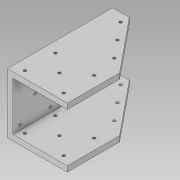
# Autodesk Inventor part: complex_cube
Saved by Autodesk Inventor 2017 (Build 210142000, 142)
## iProperties
Part Number: complex_cube
Material: Generisch
Document SubType Name: Modeling
Designer: Max
Density: 1 g/cm^3
Appearance: Vorgabe
Author: Max
Autodesk Inventor part; units mm, degrees
ref_plane "YZ Plane" through (0, 0, 0) normal (1, 0, 0) x (0, 1, 0)
ref_plane "XZ Plane" through (0, 0, 0) normal (0, 1, 0) x (-1, 0, 0)
ref_plane "XY Plane" through (0, 0, 0) normal (0, 0, 1) x (1, 0, 0)
sketch "Skizze1" plane through (0, 0, 0) normal (0, 1, 0) x (-1, 0, 0)
  line L0 (-27, 27) -> (27, 27)
  line L1 (27, 27) -> (27, -27)
  line L2 (27, -27) -> (-27, -27)
  line L3 (-27, -27) -> (-27, 27)
  line L4 (-27, 27) -> (27, -27) construction
  line L5 (27, 27) -> (-27, -27) construction
  point P0 (0, 0)
  dimension "d0" = 54
  dimension "d1" = 54
  constraints: 12 end point, 2 midpoint, 2 parallel, 1 horizontal, 1 perpendicular
  measures "d0" distance of L1.end L2.end
  measures "d1" distance of L0.end L1.end
extrude "Extrusion1" add sketch "Skizze1" along normal blind 95
sketch "Skizze2" plane through (27, 0, 27) normal (1, 0, 0) x (0, 0, -1)
  line L0 (5, 0) -> (49, 0)
  line L1 (49, 0) -> (49, 95)
  line L2 (49, 95) -> (5, 95)
  line L3 (5, 95) -> (5, 0)
  line L4 (0, 0) -> (0, 95) projected
  line L5 (54, 0) -> (54, 95) projected
  line L6 (54, 0) -> (0, 0) projected
  line L7 (54, 0) -> (54, 95) projected
  line L8 (0, 95) -> (54, 95) projected
  line L9 (0, 0) -> (0, 95) projected
  line L10 (0, 95) -> (54, 95) projected
  line L11 (54, 0) -> (0, 0) projected
  point P0 (27, 0)
  dimension "d4" = 5
  dimension "d5" = 5
  constraints: 8 end point, 2 parallel, 2 point on line, 1 horizontal, 1 perpendicular
  measures "d4" distance between parallel lines of L3 L4
  measures "d5" distance between parallel lines of L5 L1
extrude "Extrusion2" cut sketch "Skizze2" against normal blind 49 contours L3 L2 L1 L0
sketch "Skizze3" plane through (27, 0, -27) normal (0, 0, -1) x (-1, 0, 0)
  line L0 (54, 0) -> (0, 0) projected
  line L1 (54, 0) -> (54, 95) projected
  line L2 (0, 95) -> (54, 95) projected
  line L3 (0, 0) -> (0, 95) projected
  line L4 (61.4003, 122.4392) -> (0, 47.227)
  line L5 (0, 47.227) -> (39, 95)
  line L6 (39, 95) -> (33.5775, 99.4267) construction
  line L7 (33.5775, 99.4267) -> (-5.4225, 51.6538) construction
  line L8 (-5.4225, 51.6538) -> (0, 47.227) construction
  line L9 (31.8094, 54.61) -> (-25.1559, 101.1143) construction
  line L10 (27.9901, 92.5825) -> (-13.8409, 126.7317)
  line L11 (-13.8409, 126.7317) -> (-47.9901, 84.9007)
  line L12 (-47.9901, 84.9007) -> (-6.1591, 50.7515) construction
  line L13 (-6.1591, 50.7515) -> (27.9901, 92.5825) construction
  line L14 (27.9901, 92.5825) -> (-47.9901, 84.9007) construction
  line L15 (-13.8409, 126.7317) -> (-6.1591, 50.7515) construction
  line L16 (0, 95) -> (54, 95) projected
  point P0 (27, 0)
  point P1 (-10, 88.7416)
  point P2 (-10, 88.7416)
  dimension "d34" = 7
  dimension "d35" = 61.6706
  dimension "d36" = 25.8353
  dimension "d37" = 54
  dimension "d38" = 54
  dimension "d39" = 15
  dimension "d60" = 10
  constraints: 24 end point, 4 parallel, 3 midpoint, 3 perpendicular, 3 point on line, 2 collinear
  measures "d34" distance of L7.end L4.end
  measures "d35" distance of L5.end L4.end
  measures "d36" distance from line of L4.end L9
  measures "d37" distance of L11.end L12.end
  measures "d38" distance of L10.end L11.end
  measures "d39" distance of L5.end L1.end
  measures "d60" distance from line of point (-10, 88.742) L3
extrude "Extrusion3" cut sketch "Skizze3" against normal through all contours L3 L2 L4
sketch "Skizze4" plane through (27, 0, -27) normal (0, 0, -1) x (-1, 0, 0)
  line L0 (9.5, 6.25) -> (44.5, 6.25)
  line L1 (44.5, 6.25) -> (44.5, 33.75)
  line L2 (44.5, 33.75) -> (9.5, 33.75)
  line L3 (9.5, 33.75) -> (9.5, 6.25)
  line L4 (9.5, 6.25) -> (44.5, 33.75) construction
  line L5 (44.5, 6.25) -> (9.5, 33.75) construction
  line L6 (27, 0) -> (27, 60.1271) construction
  line L7 (54, 0) -> (0, 0) construction
  point P0 (27, 20)
  point P1 (27, 20)
  dimension "d11" = 35
  dimension "d12" = 27.5
  dimension "d62" = 20
  constraints: 14 end point, 3 midpoint, 2 parallel, 2 perpendicular, 1 horizontal, 1 point on line, 1 vertical
  measures "d11" distance of L1.end L2.end
  measures "d12" distance of L0.end L1.end
  measures "d62" distance from line of L7 point (27, 20)
hole "Bohrung1" at (17.5, 33.75, -27) at (-17.5, 33.75, -27) at (-17.5, 6.25, -27) at (0, 20, -27) at (17.5, 6.25, -27) direction (0, 0, 1) diameter 2.459 end up to face face through (-5.6667, 47.409, -22) facing (0, 0, 1) thread size "M3x0.5" class "6H" standard "ISO Metric profile"
sketch "Skizze5" plane through (27, 47.227, -22) normal (0.7746482, 0.6323925, 0) x (0, 0, -1)
  line L0 (-49, 0) -> (-49, 61.6706) projected
  line L1 (-44, 0) -> (-49, 0) projected
  line L2 (-44, 61.6706) -> (-44, 0) projected
  line L3 (0, 61.6706) -> (5, 61.6706) projected
  line L4 (0, 0) -> (0, 61.6706) projected
  line L5 (5, 0) -> (0, 0) projected
  line L6 (5, 61.6706) -> (5, 0) projected
  line L7 (0, 61.6706) -> (5, 61.6706) projected
  line L8 (-49, 0) -> (-49, 61.6706) projected
  line L9 (-44, 0) -> (-49, 0) projected
  line L10 (-44, 61.6706) -> (-44, 0) projected
  line L11 (-49, 61.6706) -> (-44, 61.6706) projected
  line L12 (0, 0) -> (0, 61.6706) projected
  line L13 (5, 0) -> (0, 0) projected
  line L14 (5, 61.6706) -> (5, 0) projected
  line L15 (-49, 61.6706) -> (-44, 61.6706) projected
  point P0 (127.5861, 27)
  point P1 (-46.5, 55)
  point P2 (2.5, 55)
  dimension "d41" = 2.5
  dimension "d42" = 2.5
  dimension "d43" = 55
  dimension "d44" = 55
  measures "d41" distance from line of point (2.5, 55) L6
  measures "d42" distance from line of point (-46.5, 55) L0
  measures "d43" distance from line of L1 point (-46.5, 55)
  measures "d44" distance from line of point (2.5, 55) L5
hole "Bohrung2" [suppressed]
pattern_linear "Rechteckige Anordnung1" [suppressed]
pattern_circular "Runde Anordnung1" count 3 over 180 about axis through (0, -10, 0) along (0, 1, 0) of "Bohrung1"
sketch "Skizze6" plane through (-27, 0, 27) normal (0, 0, 1) x (1, 0, 0)
  circle A0 centre (27, 20) radius 1.2295 projected
  circle A1 centre (9.5, 6.25) radius 1.2295 projected
  circle A2 centre (44.5, 6.25) radius 1.2295 projected
  circle A3 centre (9.5, 33.75) radius 1.2295 projected
  circle A4 centre (44.5, 33.75) radius 1.2295 projected
  line L0 (54, 47.227) -> (15, 95) projected
  line L1 (0, 95) -> (15, 95) projected
  line L2 (0, 0) -> (0, 95) projected
  line L3 (54, 0) -> (0, 0) projected
  line L4 (54, 0) -> (54, 47.227) projected
  line L5 (5, 95) -> (5, 0) construction
  line L6 (15, 95) -> (-19.3701, 66.9416) construction
  line L7 (54, 47.227) -> (15, 95) construction
  point P0 (27, 0)
  point P1 (27.4648, 71.8248)
  dimension "d48" = 5
  dimension "d49" = 25.8353
  dimension "d61" = 61.6706
  constraints: 2 end point, 1 perpendicular
  measures "d48" distance from line of L0 point (27.465, 71.825)
  measures "d49" distance from line of L6 point (27.465, 71.825)
  measures "d61" distance of L0.start L0.end
hole "Bohrung3" at (0.4648, 71.8248, 27) direction (0, 0, -1) diameter 2.459 end through all thread size "M3x0.5" class "6H" standard "ISO Metric profile"
pattern_linear "Rechteckige Anordnung2" count 3 spacing 20 along (-0.6323925, 0.7746482, 0) of "Bohrung3" first direction both ways yes
